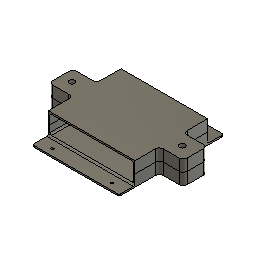
EC_MountingBracket (Autodesk Fusion 360 design; units mm, degrees)
Autodesk Fusion 360 part; units mm, degrees
sketch "Sketch1" plane through (0, 0, 0) normal (0, 1, 0) x (1, 0, 0)
  line L0 (0, 0) -> (105, 0)
  line L1 (105, 0) -> (105, 87.5)
  line L2 (105, 87.5) -> (0, 87.5)
  line L3 (0, 87.5) -> (0, 0)
  dimension "d1" = 105
  dimension "d4" = 87.5
  constraint horizontal L0
  constraint vertical L1
  constraint horizontal L2
  constraint vertical L3
  constraint coincident L0.start L3.end
  measures "d1" distance of L0.start L0.end
  measures "d4" distance of L0 L2
extrude "Extrude1" add sketch "Sketch1" along normal blind 25 makes body 1
shell "Shell1" thickness 2 outward yes removed faces 0 bodies 1
sketch "Sketch2" plane through (-2, 0, 0) normal (-1, 0, 0) x (0, 0, 1)
  line L0 (-89.5, -2) -> (2, -2)
  line L1 (2, -2) -> (2, 27)
  line L2 (2, 27) -> (-89.5, 27)
  line L3 (-89.5, 27) -> (-89.5, -2)
  line L4 (-43.75, 27) -> (-28.75, 27)
  line L5 (-28.75, 27) -> (-28.75, -2)
  line L6 (-28.75, -2) -> (-43.75, -2)
  line L7 (-43.75, 27) -> (-58.75, 27)
  line L8 (-58.75, 27) -> (-58.75, -2)
  line L9 (-58.75, -2) -> (-43.75, -2)
  dimension "d10" = 15
  dimension "d11" = 29
  constraint horizontal L4
  constraint vertical L5
  constraint horizontal L6
  constraint midpoint L2 L4.start
  constraint horizontal L7
  constraint vertical L8
  constraint horizontal L9
  measures "d10" distance of L4.start L4.end
  measures "d11" distance of L4.start L6.end
extrude "Extrude2" add sketch "Sketch2" along normal blind 30 contours L0 L2 L4 L5 L6 L7 L8 L9 bodies 1
sketch "Sketch3" plane through (107, 0, 0) normal (1, 0, 0) x (0, 0, -1)
  line L0 (-2, -2) -> (89.5, -2)
  line L1 (89.5, -2) -> (89.5, 27)
  line L2 (89.5, 27) -> (-2, 27)
  line L3 (-2, 27) -> (-2, -2)
  line L4 (43.75, 27) -> (58.75, 27)
  line L5 (58.75, 27) -> (58.75, -2)
  line L6 (58.75, -2) -> (43.75, -2)
  line L7 (43.75, 27) -> (28.75, 27)
  line L8 (28.75, 27) -> (28.75, -2)
  line L9 (28.75, -2) -> (43.75, -2)
  dimension "d14" = 15
  dimension "d15" = 29
  dimension "d16" = 29
  constraint horizontal L4
  constraint vertical L5
  constraint horizontal L6
  constraint midpoint L2 L4.start
  constraint horizontal L7
  constraint vertical L8
  constraint horizontal L9
  measures "d14" distance of L4.start L4.end
  measures "d15" distance of L4.start L6.end
  measures "d16" distance of L4.start L6.end
extrude "Extrude3" add sketch "Sketch3" along normal blind 15 contours L0 L2 L4 L5 L6 L7 L8 L9 bodies 1
extrude "Extrude4" add 1 faces at (122, 7.6667, -38.75) along direction (1, 0, 0) blind 15 on bodies 1 bodies 1
hole "Hole1" at (120.5074, -2, -43.9648) direction (0, 1, 0) diameter 7 depth 30 tip angle 180 counterbore diameter 13.5 counterbore depth 5 bodies 1
hole "Hole2" at (-18.5408, -2, -44.3993) direction (0, 1, 0) diameter 7 depth 30 tip angle 180 counterbore diameter 13.5 counterbore depth 5 bodies 1
fillet "Fillet1" radius 5 1 edges at (-2, 12.5, -58.75) on bodies 1
fillet "Fillet2" radius 5 1 edges at (-32, 12.5, -58.75) on bodies 1
fillet "Fillet3" radius 5 1 edges at (-2, 12.5, -28.75) on bodies 1
fillet "Fillet4" radius 5 1 edges at (-32, 12.5, -28.75) on bodies 1
fillet "Fillet5" radius 5 4 edges at (137, 12.5, -58.75) (107, 12.5, -58.75) (137, 12.5, -28.75) (107, 12.5, -28.75) on bodies 1
sketch "Sketch4" plane through (0, 0, -89.5) normal (0, 0, -1) x (-1, 0, 0)
  line L0 (-107, -2) -> (2, -2)
  line L1 (2, -2) -> (2, 27)
  line L2 (2, 27) -> (-107, 27)
  line L3 (-107, 27) -> (-107, -2)
  line L4 (-107, -2) -> (2, -2)
  line L5 (2, -2) -> (2, 0)
  line L6 (2, 0) -> (-107, 0)
  line L7 (-107, 0) -> (-107, -2)
  dimension "d41" = 2
  constraint horizontal L4
  constraint vertical L5
  constraint horizontal L6
  constraint vertical L7
  constraint coincident L0.start L3.end
  measures "d41" distance of L0.start L6.end
extrude "Extrude5" add sketch "Sketch4" along normal blind 20 contours L0 L1 L3 L4 L5 L6 L7 bodies 1
fillet "Fillet6" radius 2 1 edges at (52.5, 0, -89.5) on bodies 1
fillet "Fillet7" radius 2 1 edges at (107, -1, -109.5) on bodies 1
fillet "Fillet8" radius 2 1 edges at (-2, -1, -109.5) on bodies 1
sketch "Sketch5" plane through (0, 0, 2) normal (0, 0, 1) x (1, 0, 0)
  line L0 (-2, -2) -> (107, -2)
  line L1 (107, -2) -> (107, 27)
  line L2 (107, 27) -> (-2, 27)
  line L3 (-2, 27) -> (-2, -2)
  line L4 (-2, -2) -> (107, -2)
  line L5 (107, -2) -> (107, 0)
  line L6 (107, 0) -> (-2, 0)
  line L7 (-2, 0) -> (-2, -2)
  dimension "d50" = 2
  constraint horizontal L4
  constraint vertical L5
  constraint horizontal L6
  constraint vertical L7
  constraint coincident L0.start L3.end
  measures "d50" distance of L0.start L6.end
extrude "Extrude6" add sketch "Sketch5" along normal blind 20 contours L0 L1 L3 L4 L5 L6 L7 bodies 1
fillet "Fillet9" radius 2 1 edges at (52.5, 0, 2) on bodies 1
fillet "Fillet10" radius 2 1 edges at (-2, -1, 22) on bodies 1
fillet "Fillet11" radius 2 1 edges at (107, -1, 22) on bodies 1
hole "Hole3" at (13.9298, 0, -100.4305) direction (0, -1, 0) diameter 3 depth 2 tip angle 180 bodies 1
hole "Hole4" at (90.5038, 0, -100.4511) direction (0, -1, 0) diameter 3 depth 2 tip angle 180 bodies 1
hole "Hole5" at (15.1326, 0, 13.9271) direction (0, -1, 0) diameter 3 depth 2 tip angle 180 bodies 1
hole "Hole6" at (89.8518, 0, 13.7142) direction (0, -1, 0) diameter 3 depth 2 tip angle 180 bodies 1
ref_plane "WorkPlane1" through (52.5, 12.5, -43.75) normal (0, -1, 0) x (-1, 0, 0)
split "Split1" by plane through (52.5, 12.5, -43.75) normal (0, -1, 0) bodies 1 makes body 2 at (64.6351, -2, -12.1242)
extrude "Extrude7" add 1 faces at (35, 0, -58.3333) along direction (0, 1, 0) blind 2 on bodies 2 bodies 2
sketch "Sketch6" plane through (0, 2, 0) normal (0, 1, 0) x (-1, 0, 0)
  line L0 (0, -87.5) -> (0, 0)
  line L1 (0, 0) -> (-105, 0)
  line L2 (-105, 0) -> (-105, -87.5)
  line L3 (-105, -87.5) -> (0, -87.5)
  line L4 (0, -87.5) -> (-105, -87.5) construction
  line L5 (-105, -87.5) -> (-105, 0) construction
  line L6 (-105, 0) -> (0, 0) construction
  line L7 (0, 0) -> (0, -87.5) construction
  line L8 (0, -43.75) -> (-105, -43.75) construction
  line L9 (-52.5, -87.5) -> (-52.5, -40) construction
  line L10 (-52.5, -40) -> (-52.5, 0) construction
  line L11 (-27.8857, -87.5) -> (-27.8857, -49.5) construction
  line L12 (0, -49.5) -> (-12, -49.5) construction
  line L13 (-105, -49.5) -> (-93, -49.5) construction
  line L14 (-52.5, -87.5) -> (-52.5, -75.5) construction
  circle A0 centre (-12, -49.5) radius 2
  circle A1 centre (-52.5, -75.5) radius 2
  circle A2 centre (-93, -49.5) radius 2
  circle A3 centre (-12, -49.5) radius 3.5
  circle A4 centre (-52.5, -75.5) radius 3.5
  circle A5 centre (-93, -49.5) radius 3.5
  dimension "d73" = 38
  dimension "d74" = 12
  dimension "d75" = 12
  dimension "d76" = 12
  dimension "d77" = 4
  dimension "d78" = 4
  dimension "d79" = 4
  dimension "d99" = 7
  dimension "d100" = 7
  dimension "d101" = 7
  constraint horizontal L4
  constraint vertical L5
  constraint horizontal L6
  constraint vertical L7
  constraint coincident L1.end L2.start
  constraint coincident L0.start L3.end
  constraint midpoint L7 L8.start
  constraint midpoint L5 L8.end
  constraint midpoint L4 L9.start
  constraint perpendicular L4 L9
  constraint midpoint L1 L10.end
  constraint coincident L4 L11.start
  constraint perpendicular L4 L11
  constraint coincident L7 L12.start
  constraint perpendicular L7 L12
  constraint coincident L5 L13.start
  constraint perpendicular L5 L13
  constraint perpendicular L4 L14
  constraint coincident L12.end A0.centre
  constraint coincident L14.end A1.centre
  constraint coincident L13.end A2.centre
  constraint concentric A0 A3
  constraint concentric A1 A4
  constraint concentric A2 A5
  measures "d73" distance of L11.start L11.end
  measures "d74" distance of L12.start L12.end
  measures "d75" distance of L13.start L13.end
  measures "d76" distance of L9.start L14.end
  measures "d77" diameter of A0
  measures "d78" diameter of A1
  measures "d79" diameter of A2
  measures "d99" diameter of A3
  measures "d100" diameter of A4
  measures "d101" diameter of A5
extrude "Extrude8" cut sketch "Sketch6" against normal up to surface (4 mm away) contours A0 bodies 2
extrude "Extrude9" cut sketch "Sketch6" against normal up to surface (4 mm away) contours A1 | A2 bodies 2
sketch "Sketch7" plane through (0, -2, 0) normal (0, -1, 0) x (1, 0, 0)
  circle A0 centre (52.5, -75.5) radius 2
  circle A1 centre (93, -49.5) radius 2
  circle A2 centre (12, -49.5) radius 2
  circle A3 centre (89.8518, 13.7142) radius 1.5
  circle A4 centre (15.1326, 13.9271) radius 1.5
  circle A5 centre (90.5038, -100.4511) radius 1.5
  circle A6 centre (13.9298, -100.4305) radius 1.5
  arc A7 (107, 20) -> (105, 22) centre (105, 20) ccw
  line L0 (105, 22) -> (0, 22)
  arc A8 (0, 22) -> (-2, 20) centre (0, 20) ccw
  line L1 (-2, 20) -> (-2, -23.75)
  arc A9 (-7, -28.75) -> (-2, -23.75) centre (-7, -23.75) ccw
  line L2 (-7, -28.75) -> (-27, -28.75)
  arc A10 (-27, -28.75) -> (-32, -33.75) centre (-27, -33.75) ccw
  line L3 (-32, -33.75) -> (-32, -53.75)
  arc A11 (-32, -53.75) -> (-27, -58.75) centre (-27, -53.75) ccw
  line L4 (-27, -58.75) -> (-7, -58.75)
  arc A12 (-2, -63.75) -> (-7, -58.75) centre (-7, -63.75) ccw
  line L5 (-2, -63.75) -> (-2, -107.5)
  arc A13 (-2, -107.5) -> (0, -109.5) centre (0, -107.5) ccw
  line L6 (0, -109.5) -> (105, -109.5)
  arc A14 (105, -109.5) -> (107, -107.5) centre (105, -107.5) ccw
  line L7 (107, -107.5) -> (107, -63.75)
  arc A15 (112, -58.75) -> (107, -63.75) centre (112, -63.75) ccw
  line L8 (112, -58.75) -> (132, -58.75)
  arc A16 (132, -58.75) -> (137, -53.75) centre (132, -53.75) ccw
  line L9 (137, -53.75) -> (137, -33.75)
  arc A17 (137, -33.75) -> (132, -28.75) centre (132, -33.75) ccw
  line L10 (132, -28.75) -> (112, -28.75)
  arc A18 (107, -23.75) -> (112, -28.75) centre (112, -23.75) ccw
  line L11 (107, -23.75) -> (107, 20)
  circle A19 centre (-18.5408, -44.3993) radius 6.75
  circle A20 centre (120.5074, -43.9648) radius 6.75
  circle A21 centre (12, -49.5) radius 3.5
  circle A22 centre (93, -49.5) radius 3.5
  circle A23 centre (52.5, -75.5) radius 3.5
  dimension "d84" = 7
  dimension "d85" = 7
  dimension "d86" = 7
  constraint concentric A2 A21
  constraint concentric A1 A22
  constraint concentric A0 A23
  measures "d84" diameter of A21
  measures "d85" diameter of A22
  measures "d86" diameter of A23
extrude "Extrude10" cut sketch "Sketch7" against normal blind 2 contours A21 | A23 bodies 2
extrude "Extrude11" cut sketch "Sketch7" against normal blind 2 contours A22 bodies 2
sketch "Sketch8" plane through (0, 12.5, 0) normal (0, 1, 0) x (-1, 0, 0)
  line L0 (0, -87.5) -> (-105, -87.5)
  line L1 (-105, -87.5) -> (-105, 0)
  line L2 (-105, 0) -> (0, 0)
  line L3 (0, 0) -> (0, -87.5)
  circle A0 centre (-120.5074, -43.9648) radius 3.5
  circle A1 centre (18.5408, -44.3993) radius 3.5
  arc A2 (7, -58.75) -> (2, -63.75) centre (7, -63.75) ccw
  line L4 (7, -58.75) -> (27, -58.75)
  arc A3 (27, -58.75) -> (32, -53.75) centre (27, -53.75) ccw
  line L5 (32, -53.75) -> (32, -33.75)
  arc A4 (32, -33.75) -> (27, -28.75) centre (27, -33.75) ccw
  line L6 (27, -28.75) -> (7, -28.75)
  arc A5 (2, -23.75) -> (7, -28.75) centre (7, -23.75) ccw
  line L7 (2, -23.75) -> (2, 2)
  line L8 (2, 2) -> (-107, 2)
  line L9 (-107, 2) -> (-107, -23.75)
  arc A6 (-112, -28.75) -> (-107, -23.75) centre (-112, -23.75) ccw
  line L10 (-112, -28.75) -> (-132, -28.75)
  arc A7 (-132, -28.75) -> (-137, -33.75) centre (-132, -33.75) ccw
  line L11 (-137, -33.75) -> (-137, -53.75)
  arc A8 (-137, -53.75) -> (-132, -58.75) centre (-132, -53.75) ccw
  line L12 (-132, -58.75) -> (-112, -58.75)
  arc A9 (-107, -63.75) -> (-112, -58.75) centre (-112, -63.75) ccw
  line L13 (-107, -63.75) -> (-107, -89.5)
  line L14 (-107, -89.5) -> (2, -89.5)
  line L15 (2, -89.5) -> (2, -63.75)
  line L16 (0, 0) -> (0, 2)
  line L17 (-105, 0) -> (-105, 2)
  line L18 (0, -87.5) -> (0, -89.5)
  line L19 (-105, -87.5) -> (-105, -89.5)
  constraint coincident L2.end L3.start
  constraint coincident L8 L16.end
  constraint perpendicular L8 L16
  constraint coincident L1.end L2.start
  constraint coincident L8 L17.end
  constraint perpendicular L8 L17
  constraint coincident L0.start L3.end
  constraint coincident L14 L18.end
  constraint perpendicular L14 L18
  constraint coincident L0.end L1.start
  constraint coincident L14 L19.end
  constraint perpendicular L14 L19
extrude "Extrude13" cut sketch "Sketch8" against normal up to surface (10.5 mm away) contours L0 L14 L18 L19 bodies 2
extrude "Extrude12" cut sketch "Sketch8" against normal up to surface (10.5 mm away) contours L2 L8 L16 L17 bodies 2
fillet "Fillet12" radius 2 1 edges at (0, 2, -43.75) on bodies 2
fillet "Fillet13" radius 2 1 edges at (105, 2, -43.75) on bodies 2
extrude "Extrude14" add sketch "Sketch6" along normal blind 1 contours A3 | A4 | A5 bodies 2
sketch "Sketch9" plane through (0, 12.5, 0) normal (0, -1, 0) x (1, 0, 0)
  arc A0 (-2, -63.75) -> (-7, -58.75) centre (-7, -63.75) ccw
  line L0 (-2, -63.75) -> (-2, -89.5)
  line L1 (-2, -89.5) -> (107, -89.5)
  line L2 (107, -89.5) -> (107, -63.75)
  arc A1 (112, -58.75) -> (107, -63.75) centre (112, -63.75) ccw
  line L3 (112, -58.75) -> (132, -58.75)
  arc A2 (132, -58.75) -> (137, -53.75) centre (132, -53.75) ccw
  line L4 (137, -53.75) -> (137, -33.75)
  arc A3 (137, -33.75) -> (132, -28.75) centre (132, -33.75) ccw
  line L5 (132, -28.75) -> (112, -28.75)
  arc A4 (107, -23.75) -> (112, -28.75) centre (112, -23.75) ccw
  line L6 (107, -23.75) -> (107, 2)
  line L7 (107, 2) -> (-2, 2)
  line L8 (-2, 2) -> (-2, -23.75)
  arc A5 (-7, -28.75) -> (-2, -23.75) centre (-7, -23.75) ccw
  line L9 (-7, -28.75) -> (-27, -28.75)
  arc A6 (-27, -28.75) -> (-32, -33.75) centre (-27, -33.75) ccw
  line L10 (-32, -33.75) -> (-32, -53.75)
  arc A7 (-32, -53.75) -> (-27, -58.75) centre (-27, -53.75) ccw
  line L11 (-27, -58.75) -> (-7, -58.75)
  circle A8 centre (-18.5408, -44.3993) radius 3.5
  circle A9 centre (120.5074, -43.9648) radius 3.5
  line L12 (105, -87.5) -> (0, -87.5)
  line L13 (0, -87.5) -> (0, 0)
  line L14 (0, 0) -> (105, 0)
  line L15 (105, 0) -> (105, -87.5)
  line L16 (105, -87.5) -> (105, -89.5)
  line L17 (0, -87.5) -> (0, -89.5)
  line L18 (0, 0) -> (0, 2)
  line L19 (105, 0) -> (105, 2)
  constraint coincident L12.start L15.end
  constraint coincident L1 L16.end
  constraint perpendicular L1 L16
  constraint coincident L12.end L13.start
  constraint coincident L1 L17.end
  constraint perpendicular L1 L17
  constraint coincident L13.end L14.start
  constraint coincident L7 L18.end
  constraint perpendicular L7 L18
  constraint coincident L14.end L15.start
  constraint coincident L7 L19.end
  constraint perpendicular L7 L19
extrude "Extrude15" cut sketch "Sketch9" against normal up to surface (12.5 mm away) contours L7 L14 L18 L19 bodies 1
extrude "Extrude16" cut sketch "Sketch9" against normal up to surface (12.5 mm away) contours L1 L12 L16 L17 bodies 1
fillet "Fillet14" radius 2 1 edges at (105, 25, -43.75) on bodies 1
fillet "Fillet15" radius 2 1 edges at (0, 25, -43.75) on bodies 1
equation "d1 = LEN"
equation "LEN = 105 mm"
equation "WID = 87.5 mm"
equation "d4 = WID"
equation "HGT = 25 mm"
equation "d6 = HGT"
equation "THK = 2 mm"
equation "d9 = THK"
equation "d102 = THK / 2"
named bodies: "TOP_LID", "BOTTOM"
